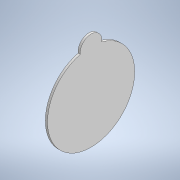
# Autodesk Inventor part: knee_drive_plate
Saved by Autodesk Inventor 2022.5 (Build 265521000, 521)
## iProperties
Created: 2024-06-27
Part Number: knee_drive_plate
Material: 一般
Document SubType Name: Modeling
Designer: gakut
Density: 1 g/cm^3
Appearance: 既定
Author: gakut
Autodesk Inventor part; units mm, degrees
ref_plane "YZ Plane" through (0, 0, 0) normal (1, 0, 0) x (0, 1, 0)
ref_plane "XZ Plane" through (0, 0, 0) normal (0, 1, 0) x (-1, 0, 0)
ref_plane "XY Plane" through (0, 0, 0) normal (0, 0, 1) x (1, 0, 0)
sketch "スケッチ1" plane through (0, 0, 0) normal (1, 0, 0) x (0, 1, 0)
  circle A0 centre (0, 0) radius 20
  circle A1 centre (20, 0) radius 5
  point P0 (19.375, 4.9608)
  point P1 (19.375, -4.9608)
  dimension "d0" = 40
  dimension "d1" = 20
  dimension "d2" = 10
  constraints: 1 centre point, 1 coincident, 1 horizontal alignment, 2 other
  measures "d1" distance of point (0, 0) A1.centre
  measures "d2" diameter of A1
extrude "押し出し1" add sketch "スケッチ1" along normal blind 1
